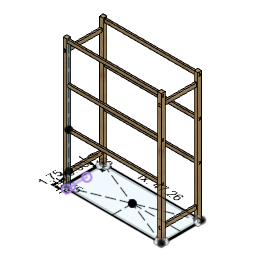
Hydroponic Frame v10 (Autodesk Fusion 360 design; units mm, degrees)
Autodesk Fusion 360 part; units mm, degrees
sketch "footprint" plane through (0, 0, 0) normal (0, 1, 0) x (1, 0, 0)
  line L0 (600.2, -241.3) -> (-600.2, -241.3)
  line L1 (-600.2, -241.3) -> (-600.2, 241.3)
  line L2 (-600.2, 241.3) -> (600.2, 241.3)
  line L3 (600.2, 241.3) -> (600.2, -241.3)
  line L4 (600.2, -241.3) -> (-600.2, 241.3) construction
  line L5 (-600.2, -241.3) -> (600.2, 241.3) construction
  line L6 (-587.5, 241.3) -> (-587.5, -241.3)
  line L7 (-587.5, -195.202) -> (-543.05, -195.202)
  line L8 (-543.05, -195.202) -> (-543.05, -239.652)
  line L9 (-543.05, -239.652) -> (-587.5, -239.652)
  line L10 (-587.5, -239.652) -> (-587.5, -195.202)
  line L11 (0, 0) -> (600.2, 0) construction
  line L12 (600.2, 0) -> (600.2, -241.3) construction
  line L13 (600.2, -241.3) -> (0, -241.3) construction
  line L14 (0, -241.3) -> (0, 0) construction
  line L15 (587.5, 241.3) -> (587.5, -241.3)
  line L16 (587.5, -195.202) -> (543.05, -195.202)
  line L17 (543.05, -195.202) -> (543.05, -239.652)
  line L18 (-587.5, 195.202) -> (-543.05, 195.202)
  line L19 (543.05, 195.202) -> (543.05, 239.652)
  line L20 (587.5, 195.202) -> (543.05, 195.202)
  line L21 (-543.05, 195.202) -> (-543.05, 239.652)
  dimension "d10" = 1200.3999
  dimension "d11" = 482.6
  dimension "d12" = 12.7
  dimension "d13" = 44.45
  dimension "d14" = 44.45
  constraint horizontal L0
  constraint perpendicular L0 L1
  constraint parallel L0 L2
  constraint parallel L1 L3
  constraint coincident L4 L11.start
  constraint coincident L5 L11.start
  constraint coincident L11.start L14.end
  constraint coincident L2 L6.start
  constraint coincident L0 L6.end
  constraint perpendicular L0 L6
  constraint horizontal L7
  constraint vertical L8
  constraint horizontal L9
  constraint vertical L10
  constraint coincident L6 L7.start
  constraint horizontal L11
  constraint vertical L12
  constraint horizontal L13
  constraint vertical L14
  constraint symmetric L6.start L14 L15.start
  constraint symmetric L6.end L14 L15.end
  constraint symmetric L7.start L14 L16.start
  constraint symmetric L7.end L14 L16.end
  constraint symmetric L8.end L14 L17.end
  constraint symmetric L7.start L11 L18.start
  constraint symmetric L7.end L11 L18.end
  constraint symmetric L8.end L11 L21.end
  constraint symmetric L11 L16.start L20.start
  constraint symmetric L11 L16.end L19.start
  constraint symmetric L11 L17.end L19.end
  measures "d10" distance of L1.end L2.end
  measures "d11" distance of L0.end L1.end
  measures "d12" distance of L1 L6
  measures "d13" distance of L7.start L7.end
  measures "d14" distance of L7.start L9.end
extrude "Extrude1" add sketch "footprint" along normal blind 1549.4 contours L6 L7 L8 L9 L10 makes body 1 in component "leg 1"
sketch "Sketch2" plane through (0, 0, 0) normal (0, 0, 1) x (1, 0, 0)
sketch "rail" plane through (0, 0, 195.202) normal (0, 0, -1) x (-1, 0, 0)
  line L0 (543.05, 0) -> (587.5, 0)
  line L1 (587.5, 0) -> (587.5, 1549.4)
  line L2 (587.5, 1549.4) -> (543.05, 1549.4)
  line L3 (543.05, 1549.4) -> (543.05, 0)
  line L4 (574.8, 127) -> (555.75, 127)
  line L5 (555.75, 127) -> (555.75, 171.45)
  line L6 (555.75, 171.45) -> (574.8, 171.45)
  line L7 (574.8, 171.45) -> (574.8, 127)
  line L8 (574.8, 127) -> (555.75, 171.45) construction
  line L9 (555.75, 127) -> (574.8, 171.45) construction
  line L10 (571.6504, 133.35) -> (558.8996, 133.35)
  line L11 (558.8996, 133.35) -> (558.8996, 165.1)
  line L12 (558.8996, 165.1) -> (571.6504, 165.1)
  line L13 (571.6504, 165.1) -> (571.6504, 133.35)
  line L14 (571.6504, 133.35) -> (558.8996, 165.1) construction
  line L15 (558.8996, 133.35) -> (571.6504, 165.1) construction
  point P0 (565.275, 149.225)
  point P1 (565.275, 149.225)
  point P2 (543.05, 0)
  dimension "d20" = 19.05
  dimension "d21" = 44.45
  dimension "d22" = 3.1496
  dimension "d23" = 6.35
  dimension "d30" = 127
  dimension "d31" = 12.7
  constraint horizontal L4
  constraint parallel L4 L6
  constraint parallel L5 L7
  constraint coincident L8 P1
  constraint coincident L9 P1
  constraint horizontal L10
  constraint perpendicular L10 L11
  constraint parallel L10 L12
  constraint parallel L11 L13
  constraint coincident L14 P1
  constraint coincident L15 P1
  constraint coincident P1 P0
  measures "d20" distance of L5.end L6.end
  measures "d21" distance of L4.start L6.end
  measures "d22" distance of L7 L13
  measures "d23" distance of L6 L12
  measures "d30" distance of L4 P2
  measures "d31" distance of L1 L7
extrude "Extrude1'" add sketch "rail" along normal up to surface (482.6 mm away) from surface at -46.098 separate body contours L10 L11 L12 L13 makes body 2 in component "short rail"
extrude "Extrude2" add sketch "rail" along normal up to surface (390.4039 mm away) contours L4 L5 L6 L7 bodies 2 in component "short rail"
sketch "long rail" plane through (-543.05, 0, 0) normal (1, 0, 0) x (0, 0, -1)
  line L0 (-239.652, 0) -> (-195.202, 0)
  line L1 (-195.202, 0) -> (-195.202, 1549.4)
  line L2 (-195.202, 1549.4) -> (-239.652, 1549.4)
  line L3 (-239.652, 1549.4) -> (-239.652, 0)
  line L4 (-217.427, 0) -> (-217.427, 1549.4) construction
  line L5 (-207.902, 584.2) -> (-226.952, 584.2)
  line L6 (-226.952, 584.2) -> (-226.952, 622.6073)
  line L7 (-226.952, 622.6073) -> (-207.902, 622.6073)
  line L8 (-207.902, 622.6073) -> (-207.902, 584.2)
  line L9 (-207.902, 584.2) -> (-226.952, 622.6073) construction
  line L10 (-226.952, 584.2) -> (-207.902, 622.6073) construction
  line L11 (-211.0516, 590.55) -> (-223.8024, 590.55)
  line L12 (-223.8024, 590.55) -> (-223.8024, 616.2573)
  line L13 (-223.8024, 616.2573) -> (-211.0516, 616.2573)
  line L14 (-211.0516, 616.2573) -> (-211.0516, 590.55)
  line L15 (-211.0516, 590.55) -> (-223.8024, 616.2573) construction
  line L16 (-223.8024, 590.55) -> (-211.0516, 616.2573) construction
  line L17 (0, 0) -> (-241.3, 0)
  point P0 (-217.427, 603.4036)
  point P1 (-217.427, 603.4036)
  dimension "d36" = 19.05
  dimension "d37" = 6.35
  dimension "d38" = 3.1496
  dimension "d39" = 584.2
  constraint midpoint L0 L4.start
  constraint midpoint L2 L4.end
  constraint horizontal L5
  constraint perpendicular L5 L6
  constraint parallel L5 L7
  constraint parallel L6 L8
  constraint coincident L9 P1
  constraint coincident L10 P1
  constraint coincident L4 P1
  constraint horizontal L11
  constraint perpendicular L11 L12
  constraint parallel L11 L13
  constraint parallel L12 L14
  constraint coincident L15 P1
  constraint coincident L16 P1
  constraint coincident L9 L11.start
  constraint coincident P1 P0
  measures "d36" distance of L6.end L7.end
  measures "d37" distance of L7 L13
  measures "d38" distance of L8 L14
  measures "d39" distance of L5 L17
extrude "Extrude1''" add sketch "long rail" along normal up to surface (1130.5499 mm away) separate body contours L11 L12 L13 L14 makes body 3 in component "long rail"
extrude "Extrude2'" add sketch "long rail" along normal up to surface (1086.0999 mm away) contours L5 L6 L7 L8 bodies 3 in component "long rail"
pattern_linear "R-Pattern1" count 3 spacing 457.2 along (0, 1, 0) of bodies 3 makes body 4 at (-181.0167, 1054.2024, 226.952) makes body 5 at (-181.0167, 1511.4024, 226.952) in component "long rail"
pattern_linear "R-Pattern1'" count 2 spacing 1270 along (0, 1, 0) of bodies 2 makes body 6 in component "short rail"
mirror "MirrorComponent1" about plane through (0, 0, 0) normal (0, 0, 1) of bodies 2 6 makes body 7 at (-555.75, 141.8167, 65.0673) makes body 8 at (-555.75, 1411.8167, 65.0673) in component "short rail(Mirror)"
mirror "MirrorComponent1'" about plane through (0, 0, 0) normal (0, 0, 1) of bodies 1 makes body 9 in component "leg 1(Mirror)"
mirror "MirrorComponent2" about plane through (0, 0, 0) normal (0, 0, 1) of bodies 3 4 5 makes body 10 at (-181.0167, 597.0024, -226.952) makes body 11 at (-181.0167, 1054.2024, -226.952) makes body 12 at (-181.0167, 1511.4024, -226.952) in component "long rail(Mirror)"
mirror "MirrorComponent2'" about plane through (0, 0, 0) normal (0, 0, 1) of bodies 1 makes body 13 in component "leg 1(Mirror) (1)"
mirror "MirrorComponent2''" about plane through (0, 0, 0) normal (0, 0, 1) of bodies 9 makes body 14 in component "leg 1(Mirror)(Mirror)"
component "leg 1" placed x (1, 0, 0) y (0, 1, 0) z (0, 0, 1) at (0, 0, 0)
component "short rail" placed x (1, 0, 0) y (0, 1, 0) z (0, 0, 1) at (0, 0, 0)
component "long rail" placed x (1, 0, 0) y (0, 1, 0) z (0, 0, 1) at (0, 0, 0)
component "leg 1(Mirror)" placed x (-1, 0, 0) y (0, 1, 0) z (0, 0, -1) at (0, 0, 0)
component "short rail(Mirror)" placed x (-1, 0, 0) y (0, 1, 0) z (0, 0, -1) at (0, 0, 0)
component "leg 1(Mirror) (1)" placed x (1, 0, 0) y (0, 1, 0) z (0, 0, 1) at (0, 0, 0)
component "long rail(Mirror)" placed x (1, 0, 0) y (0, 1, 0) z (0, 0, 1) at (0, 0, 0)
component "leg 1(Mirror)(Mirror)" placed x (-1, 0, 0) y (0, 1, 0) z (0, 0, -1) at (0, 0, 0)
equation "thiness = 0.728 in"
equation "height = 61 in"
equation "width = 23.622 in"
equation "length = 46.25984 in"
equation "bitSize = 0.25 in"
equation "bitSize125 = 0.125 in"
equation "crossBeam = 1.5 in"
equation "d10 = length + 1 in"
equation "d15 = height"
equation "firstLay = 20 in"
equation "first_floor = 23 in"
equation "second_floor = 20 in"
equation "third_floor = 20 in"
equation "d39 = first_floor"
